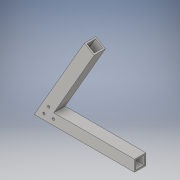
# Autodesk Inventor part: 60DegreeAlumTubing
Saved by Autodesk Inventor 2016 SP1 (Build 200210100, 210)
## iProperties
Created: 2016-01-25
Part Number: 60DegreeAlumTubing
Material: Generic
Document SubType Name: Modeling
Designer: steele
Density: 1 g/cm^3
Appearance: Default
Author: steele
Autodesk Inventor part; units mm, degrees
ref_plane "YZ Plane" through (0, 0, 0) normal (1, 0, 0) x (0, 1, 0)
ref_plane "XZ Plane" through (0, 0, 0) normal (0, 1, 0) x (-1, 0, 0)
ref_plane "XY Plane" through (0, 0, 0) normal (0, 0, 1) x (1, 0, 0)
sketch "Sketch1" plane through (0, 0, 0) normal (0, 0, 1) x (1, 0, 0)
  line L0 (0, 0) -> (-203.2, 0)
  line L1 (-203.2, 0) -> (-101.6, 175.9764)
  dimension "d0" = 60
  dimension "d1" = 203.2
  constraints: 4 end point, 1 equal length, 1 horizontal
  measures "d0" angle of L1 L0
  measures "d1" distance of L0.start L0.end
sketch "Sketch2" plane through (0, 0, 0) normal (1, 0, 0) x (0, 1, 0)
  line L0 (-12.7, 12.7) -> (-12.7, -12.7)
  line L1 (-12.7, -12.7) -> (12.7, -12.7)
  line L2 (12.7, -12.7) -> (12.7, 12.7)
  line L3 (12.7, 12.7) -> (-12.7, 12.7)
  line L4 (-12.7, 12.7) -> (12.7, -12.7) construction
  line L5 (-12.7, -12.7) -> (12.7, 12.7) construction
  line L6 (-9.525, 9.525) -> (-9.525, -9.525)
  line L7 (-9.525, -9.525) -> (9.525, -9.525)
  line L8 (9.525, -9.525) -> (9.525, 9.525)
  line L9 (9.525, 9.525) -> (-9.525, 9.525)
  line L10 (-9.525, 9.525) -> (9.525, -9.525) construction
  line L11 (-9.525, -9.525) -> (9.525, 9.525) construction
  point P0 (0, 0)
  dimension "d2" = 25.4
  dimension "d3" = 3.175
  constraints: 24 end point, 4 midpoint, 4 parallel, 4 perpendicular, 2 vertical
  measures "d2" distance of L0.start L0.end
  measures "d3" distance between parallel lines of L0 L6
sweep "Sweep1" add profiles "Sketch2" path "Sketch1"
sketch "Sketch3" plane through (0, -12.7, 12.7) normal (0, 0, 1) x (1, 0, 0)
  line L0 (0, 0) -> (-225.197, 0) construction
  line L1 (0, 25.4) -> (-181.203, 25.4) construction
  line L2 (-225.197, 0) -> (-181.203, 25.4) construction
  circle A0 centre (-203.2, 12.7) radius 2.54
  line L3 (-112.5985, 195.0264) -> (-90.6015, 182.3264) construction
  line L4 (-191.2937, 33.3222) -> (-203.2, 12.7) construction
  line L5 (-203.2, 12.7) -> (-179.3875, 12.7) construction
  circle A1 centre (-192.5637, 31.1225) radius 2.54
  circle A2 centre (-181.9275, 12.7) radius 2.54
  point P0 (0, 12.7)
  dimension "d6" = 5.08
  dimension "d7" = 23.8125
  constraints: 6 end point, 2 point on line, 1 centre point, 1 equal length, 1 horizontal, 1 horizontal alignment, 1 midpoint, 1 perpendicular, 7 other
  measures "d6" diameter of A0
  measures "d7" distance of L4.end L5.end
extrude "Extrusion1" cut sketch "Sketch3" against normal through all
body "Solid1"
